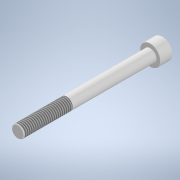
# Autodesk Inventor part: MM-MMount_to_Frame-Bolt
Saved by Autodesk Inventor 2020 (Build 240168000, 168)
## iProperties
Created: 2020-02-25
Part Number: MM-MMount_to_Frame-Bolt
Material: Generic
Document SubType Name: Modeling
Designer: Vitaliy
Density: 1 g/cm^3
Appearance: Default
Author: Vitaliy
Autodesk Inventor part; units mm, degrees
ref_plane "YZ Plane" through (0, 0, 0) normal (1, 0, 0) x (0, 1, 0)
ref_plane "XZ Plane" through (0, 0, 0) normal (0, 1, 0) x (-1, 0, 0)
ref_plane "XY Plane" through (0, 0, 0) normal (0, 0, 1) x (1, 0, 0)
sketch "Sketch1" plane through (0, 0, 0) normal (0, 0, 1) x (1, 0, 0)
  circle A0 centre (0, 0) radius 5
  dimension "d0" = 10
  constraints: 1 centre point, 1 coincident
  measures "d0" diameter of A0
extrude "Extrusion1" add sketch "Sketch1" along normal blind 6
sketch "Sketch2" plane through (0, 0, 6) normal (0, 0, 1) x (1, 0, 0)
  circle A0 centre (0, 0) radius 3
  dimension "d3" = 6
  constraints: 1 centre point, 1 coincident
  measures "d3" diameter of A0
extrude "Extrusion2" add sketch "Sketch2" along normal blind 65
thread "Thread1" size "M6x1" class "6g" standard "ISO Metric profile" length 24
fillet "Fillet2" radius 0.5 1 edges at (-3, 0, 71)
fillet "Fillet3" radius 0.2 3 edges at (-5, 0, 6) (-3, 0, 6) (-5, 0, 0)
sketch "Sketch5" plane through (0, 0, 0) normal (0, 0, -1) x (-1, 0, 0)
  line L0 (2.8868, 0) -> (1.4434, -2.5)
  line L1 (1.4434, -2.5) -> (-1.4434, -2.5)
  line L2 (-1.4434, -2.5) -> (-2.8868, 0)
  line L3 (-2.8868, 0) -> (-1.4434, 2.5)
  line L4 (-1.4434, 2.5) -> (1.4434, 2.5)
  line L5 (1.4434, 2.5) -> (2.8868, 0)
  point P0 (0, 0)
  point P1 (0, 0)
  dimension "d15" = 5
  constraints: 12 end point, 1 coincident, 13 other
  measures "d15" distance between parallel lines of L1 L4
extrude "Extrusion4" cut sketch "Sketch5" against normal blind 3.7
fillet "Fillet6" radius 0.125 6 edges at (-2.1651, -1.25, 3.7) (0, -2.5, 3.7) (0, 2.5, 3.7) (-2.1651, 1.25, 3.7) (2.1651, -1.25, 3.7) (2.1651, 1.25, 3.7)
fillet "Fillet7" radius 0.1 6 edges at (-2.1651, -1.25, 0) (0, -2.5, 0) (2.1651, -1.25, 0) (2.1651, 1.25, 0) (0, 2.5, 0) (-2.1651, 1.25, 0)
body "Solid1"
